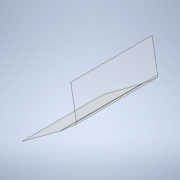
# Autodesk Inventor part: 機体ケツ防護カバーver2
Saved by Autodesk Inventor 2020.2 (Build 242310000, 310)
## iProperties
Created: 2020-05-27
Part Number: 機体ケツ防護カバーver2
Material: ポリカーボネート、クリア
Document SubType Name: Modeling
Designer: mozar
Density: 1.2 g/cm^3
Appearance: ポリカーボネート - クリア
Author: mozar
Autodesk Inventor part; units mm, degrees
ref_plane "YZ Plane" through (0, 0, 0) normal (1, 0, 0) x (0, 1, 0)
ref_plane "XZ Plane" through (0, 0, 0) normal (0, 1, 0) x (-1, 0, 0)
ref_plane "XY Plane" through (0, 0, 0) normal (0, 0, 1) x (1, 0, 0)
sketch "スケッチ1" plane through (0, 0, 0) normal (0, 0, 1) x (1, 0, 0)
  line L0 (109.2087, 3) -> (109.2087, 0)
  line L1 (109.2087, -3) -> (109.2087, 0)
  circle A0 centre (111.885, -36) radius 4
  circle A1 centre (47.8869, -85.25) radius 4
  line L2 (109.2087, 3) -> (115.8267, -35.3193)
  line L3 (116.3194, -35.2342) -> (108.7087, 8.833)
  line L4 (108.7087, 8.833) -> (108.7087, 0)
  circle A2 centre (111.885, -36) radius 4.5
  line L5 (109.2087, 3) -> (109.7014, 3.0851)
  circle A3 centre (88.5017, -43.0436) radius 13.85
  line L6 (96.7244, -54.1885) -> (50.2617, -88.4688)
  line L7 (114.4855, -39.0393) -> (97.5058, -53.5673)
  line L8 (114.8106, -39.4192) -> (97.8309, -53.9472)
  circle A4 centre (88.5017, -43.0436) radius 14.35
  line L9 (97.0213, -54.5908) -> (50.5586, -88.8711)
  line L10 (50.5586, -88.8711) -> (50.2617, -88.4688)
  point P0 (0, 0)
  dimension "d0" = 0.5
  dimension "d1" = 0.5
  dimension "d2" = 0.5
  dimension "d3" = 0.5
  dimension "d4" = 0.5
  constraints: 22 end point, 4 centre point, 4 point on circle, 4 tangent, 2 parallel, 2 perpendicular, 2 vertical, 1 point on line, 8 other
  measures "d0" distance between parallel lines of L2 L3
  measures "d1" radial gap between concentric circles of A0 A2
  measures "d2" distance between parallel lines of L7 L8
  measures "d3" radial gap between concentric circles of A3 A4
  measures "d4" distance between parallel lines of L6 L9
extrude "押し出し1" add sketch "スケッチ1" against normal blind 98.8 contours A0 L2 A2 L7 | L2 L5 L3 A2 | A2 L8 A4 L7 | A4 L6 A3 L7 | L9 L10 L6 A4 picked at (113.6675, -39.86) picked at (95.0962, -55.5046)
